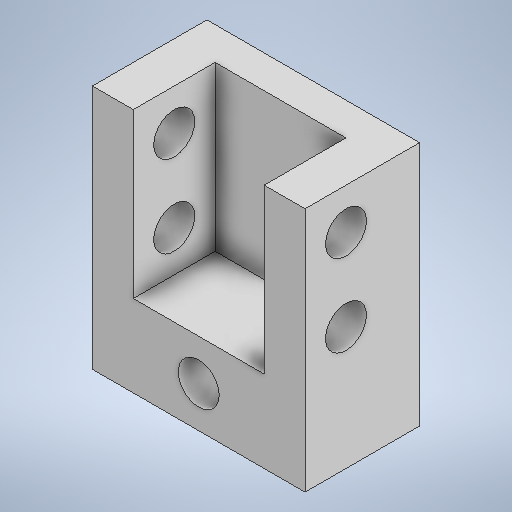
# Autodesk Inventor part: SteeringFrame
Saved by Autodesk Inventor 2025.2 (Build 292293000, 293)
## iProperties
Created: 2025-01-05
Part Number: SteeringFrame
Material: 일반
Document SubType Name: Modeling
Designer: SEON
Density: 1 g/cm^3
Appearance: 기본값
Author: SEON
Autodesk Inventor part; units mm, degrees
ref_plane "YZ Plane" through (0, 0, 0) normal (1, 0, 0) x (0, 1, 0)
ref_plane "XZ Plane" through (0, 0, 0) normal (0, 1, 0) x (-1, 0, 0)
ref_plane "XY Plane" through (0, 0, 0) normal (0, 0, 1) x (1, 0, 0)
sketch "스케치1" plane through (0, 0, 0) normal (0, 0, 1) x (1, 0, 0)
  line L0 (-13, -5) -> (13, -5)
  line L1 (13, -5) -> (13, 5)
  line L2 (13, 5) -> (-13, 5)
  line L3 (-13, 5) -> (-13, -5)
  line L4 (-13, -5) -> (13, 5) construction
  line L5 (13, -5) -> (-13, 5) construction
  circle A0 centre (0, 0) radius 2.5
  dimension "d0" = 26
  dimension "d1" = 10
  dimension "d2" = 5
  constraints: 12 end point, 2 midpoint, 2 parallel, 1 centre point, 1 coincident, 1 horizontal, 1 perpendicular
  measures "d0" distance of L1.end L2.end
  measures "d1" distance of L0.end L1.end
  measures "d2" diameter of A0
extrude "돌출1" add sketch "스케치1" along normal blind 10
sketch "스케치2" plane through (-13, 5, 0) normal (0, 1, 0) x (1, 0, 0)
  line L0 (26, 0) -> (0, 0) projected
  line L1 (26, -10) -> (0, -10) projected
  line L2 (0, 0) -> (5, 0)
  line L3 (5, 0) -> (5, -10)
  line L4 (5, -10) -> (0, -10)
  line L5 (0, -10) -> (0, 0)
  line L6 (13, 0) -> (13, -10)
  line L7 (26, 0) -> (21, 0)
  line L8 (21, 0) -> (21, -10)
  line L9 (21, -10) -> (26, -10)
  line L10 (26, -10) -> (26, 0)
  point P0 (0, -10)
  point P1 (21, 0)
  dimension "d5" = 5
  dimension "d6" = 8
  constraints: 18 end point, 4 symmetric about line, 2 parallel, 2 point on line, 1 horizontal, 1 midpoint, 1 perpendicular
  measures "d5" distance between parallel lines of L5 L3
  measures "d6" distance between parallel lines of L6 L3
extrude "돌출2" add sketch "스케치2" along normal blind 10 contours L10 L1 L8 L0 | L3 L1 L5 L0
sketch "스케치3" plane through (-13, 5, 0) normal (-1, 0, 0) x (0, 0, 1)
  circle A0 centre (5, 5) radius 2.5
  line L0 (0, 10) -> (10, 10) projected
  line L1 (10, -10) -> (10, 10) projected
  point P0 (0, -5)
  point P1 (10, 0)
  point P2 (10, 5)
  point P3 (5, 10)
  point P4 (5, 10)
  dimension "d9" = 5
  constraints: 2 midpoint, 1 centre point, 1 horizontal alignment, 1 point on line, 1 vertical alignment
  measures "d9" diameter of A0
extrude "돌출3" cut sketch "스케치3" against normal through all
ref_plane "작업 평면1" through (-13, 15, 0) normal (0, 1, 0) x (1, 0, 0)
mirror "미러1" about plane through (-10.5, 15, 5) normal (0, 1, 0) of "돌출3", "돌출2"
sketch "스케치4" plane through (0, 0, 0) normal (0, 0, -1) x (-1, 0, 0)
  line L0 (-13, 5) -> (-13, 25) projected
  line L1 (13, -5) -> (-13, -5) projected
  line L2 (-13, 25) -> (13, 25)
  line L3 (13, 25) -> (13, -5)
  line L4 (13, -5) -> (-13, -5)
  line L5 (-13, -5) -> (-13, 25)
  point P0 (0, 0)
  point P1 (13, 25)
  constraints: 8 end point, 2 parallel, 1 coincident, 1 horizontal, 1 perpendicular, 1 point on line
extrude "돌출4" add sketch "스케치4" along normal blind 4
